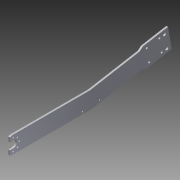
# Autodesk Inventor part: Arm_Link_1
Saved by Autodesk Inventor 2013 (Build 170138000, 138)
## iProperties
Created: 2014-05-15
Part Number: Arm_Link_1
Material: アルミニウム 6061
Document SubType Name: Modeling
Designer: andou
Density: 2.71 g/cm^3
Mass: 19.3291 g
Surface Area: 81.331 cm^2
Volume: 7.13251 cm^3
Author: andou
Autodesk Inventor part; units mm, degrees
ref_plane "YZ Plane" through (0, 0, 0) normal (1, 0, 0) x (0, 1, 0)
ref_plane "XZ Plane" through (0, 0, 0) normal (0, 1, 0) x (-1, 0, 0)
ref_plane "XY Plane" through (0, 0, 0) normal (0, 0, 1) x (1, 0, 0)
sketch "スケッチ2" plane through (0, 0, 0) normal (1, 0, 0) x (0, 1, 0)
  line L0 (0, 0) -> (-89.4689, 0)
  line L1 (-89.4689, -20) -> (1.7498, -20)
  line L2 (0, 0) -> (88.1097, 15.5361)
  line L3 (91.5826, -4.16) -> (1.7498, -20)
  arc A0 (92.1939, 15.4085) -> (88.1097, 15.5361) centre (89.8461, 5.688) ccw
  arc A1 (91.5826, -4.16) -> (95.3769, -2.6433) centre (89.8461, 5.688) ccw
  arc A2 (-93.4689, -19.1652) -> (-89.4689, -20) centre (-89.4689, -10) ccw
  arc A3 (-89.4689, 0) -> (-93.4689, -0.8348) centre (-89.4689, -10) ccw
  arc A4 (-89.4689, -14) -> (-89.4689, -6) centre (-89.4689, -10) ccw
  line L4 (-89.4689, -6) -> (-93.4689, -6)
  line L5 (-89.4689, -14) -> (-93.4689, -14)
  line L6 (-93.4689, -0.8348) -> (-93.4689, -6)
  line L7 (-93.4689, -14) -> (-93.4689, -19.1652)
  line L8 (92.1939, 15.4085) -> (93.0908, 10.3219)
  line L9 (94.48, 2.4434) -> (95.3769, -2.6433)
  line L10 (1.7498, -20) -> (0, 0)
  line L11 (93.0908, 10.3219) -> (94.48, 2.4434)
  dimension "d21" = 20
  dimension "d22" = 10
  dimension "d23" = 170
  dimension "d25" = 10
  dimension "d27" = 10
  dimension "d31" = 8
  dimension "d33" = 4
  dimension "d35" = 4
  dimension "d36" = 180
  constraints: 24 end point, 10 point on circle, 8 perpendicular, 5 centre point, 4 equal length, 3 equal radius, 2 parallel, 2 tangent, 1 coincident, 1 collinear, 1 horizontal
  measures "d21" distance between parallel lines of L0 L1
  measures "d22" distance from line of L0 A2.centre
  measures "d23" angle of L0 L2
  measures "d25" distance from line of L3 A0.centre
  measures "d27" radius of A3
  measures "d31" diameter of A4
  measures "d33" distance from line of L6 A2.centre
  measures "d35" distance from line of L8 L2.end
  measures "d36" distance of A2.centre A0.centre
extrude "押し出し1" add sketch "スケッチ2" along normal blind 2
sketch "スケッチ4" plane through (0, 0, 0) normal (-1, 0, 0) x (0, 0, 1)
  line L0 (-20, 1.7498) -> (-4.16, 91.5826) projected
  line L1 (-20, -89.4689) -> (-20, 1.7498) projected
  circle A0 centre (-17, -8.5509) radius 1
  circle A1 centre (-15.2569, 11.373) radius 1
  line L2 (-17, -8.5509) -> (-15.2569, 11.373)
  dimension "d57" = 2
  dimension "d59" = 20
  dimension "d60" = 175
  dimension "d61" = 3
  dimension "d62" = 3
  constraints: 2 centre point, 2 end point, 1 equal radius
  measures "d57" diameter of A0
  measures "d59" distance of L2.start L2.end
  measures "d60" angle of L1 L2
  measures "d61" distance from line of L1 L2.start
  measures "d62" distance from line of L0 L2.end
hole "穴2" at (0, -8.5509, -17) at (0, 11.373, -15.2569) direction (1, 0, 0) diameter 1.6 end through all
sketch "スケッチ6" plane through (2, 0, 0) normal (1, 0, 0) x (0, 0, -1)
  line L0 (20, 1.7498) -> (4.16, 91.5826) projected
  arc A0 (4.16, 91.5826) -> (2.6433, 95.3769) centre (-5.688, 89.8461) ccw projected
  line L1 (2.6433, 95.3769) -> (-15.4085, 92.1939) projected
  arc A1 (-15.4085, 92.1939) -> (-15.5361, 88.1097) centre (-5.688, 89.8461) ccw projected
  line L2 (-15.5361, 88.1097) -> (0, 0) projected
  line L3 (-10.2693, 58.2403) -> (-13.4833, 62.0705)
  line L4 (-15.4085, 92.1939) -> (-18.6927, 91.6148)
  line L5 (-18.6927, 91.6148) -> (-13.4833, 62.0705)
  line L6 (2.6433, 95.3769) -> (5.9275, 95.956)
  line L7 (5.9275, 95.956) -> (11.1369, 66.4117)
  line L8 (11.1369, 66.4117) -> (9.4268, 61.7133)
  dimension "d75" = 150
  dimension "d76" = 150
  dimension "d77" = 2.5
  dimension "d78" = 2.5
  dimension "d79" = 30
  constraints: 12 end point, 3 parallel, 2 collinear, 2 point on line
  measures "d75" angle of L2 L3
  measures "d76" angle of L0 L8
  measures "d77" distance between parallel lines of L0 L7
  measures "d78" distance between parallel lines of L2 L5
  measures "d79" distance of L4.end L3.end
extrude "押し出し2" add sketch "スケッチ6" against normal blind 2
sketch "スケッチ5" plane through (2, 0, 0) normal (1, 0, 0) x (0, 0, -1)
  line L0 (2.6433, 95.3769) -> (-15.4085, 92.1939) projected
  circle A0 centre (-13.3928, 87.4722) radius 1.5
  circle A1 centre (2.3641, 90.2505) radius 1.5
  line L1 (-13.4833, 62.0705) -> (-18.6927, 91.6148) projected
  line L2 (-18.6927, 91.6148) -> (5.9275, 95.956) projected
  line L3 (5.9275, 95.956) -> (11.1369, 66.4117) projected
  line L4 (11.1369, 66.4117) -> (9.4268, 61.7133) projected
  line L5 (9.4268, 61.7133) -> (20, 1.7498) projected
  line L6 (20, 1.7498) -> (20, -89.4689) projected
  arc A2 (19.1652, -93.4689) -> (20, -89.4689) centre (10, -89.4689) ccw projected
  line L7 (19.1652, -93.4689) -> (14, -93.4689) projected
  line L8 (14, -93.4689) -> (14, -89.4689) projected
  arc A3 (14, -89.4689) -> (6, -89.4689) centre (10, -89.4689) ccw projected
  line L9 (6, -89.4689) -> (6, -93.4689) projected
  line L10 (6, -93.4689) -> (0.8348, -93.4689) projected
  arc A4 (0, -89.4689) -> (0.8348, -93.4689) centre (10, -89.4689) ccw projected
  line L11 (0, -89.4689) -> (0, 0) projected
  line L12 (0, 0) -> (-10.2693, 58.2403) projected
  line L13 (-10.2693, 58.2403) -> (-13.4833, 62.0705) projected
  circle A5 centre (17, -8.5509) radius 0.8 projected
  circle A6 centre (15.2569, 11.373) radius 0.8 projected
  dimension "d70" = 5
  dimension "d71" = 5
  dimension "d72" = 3
  dimension "d114" = 16
  dimension "d123" = 4.5
  constraints: 2 centre point, 1 equal radius
  measures "d70" distance from line of L0 A0.centre
  measures "d71" distance from line of L0 A1.centre
  measures "d72" diameter of A1
  measures "d114" distance of A1.centre A0.centre
  measures "d123" distance from line of L1 A0.centre
hole "穴3" at (2, 87.4722, 13.3928) at (2, 90.2505, -2.3641) direction (-1, 0, 0) diameter 4 end through all
sketch "スケッチ7" plane through (2, 0, 0) normal (1, 0, 0) x (0, 0, -1)
  arc A0 (0, -89.4689) -> (0.8348, -93.4689) centre (10, -89.4689) ccw projected
  line L0 (0.8348, -93.4689) -> (6, -93.4689) projected
  circle A1 centre (3, -89.4689) radius 1
  dimension "d89" = 4
  dimension "d90" = 7
  dimension "d91" = 2
  constraints: 1 centre point
  measures "d89" distance from line of L0 A1.centre
  measures "d90" distance of A1.centre A0.centre
  measures "d91" diameter of A1
hole "穴4" at (2, -89.4689, -3) direction (-1, 0, 0) diameter 2 end through all
pattern_circular "円形状パターン3" count 5 over 180 about axis through (0, -89.4689, -10) along (-1, 0, 0) of "穴4"
sketch "スケッチ8" plane through (2, 0, 0) normal (1, 0, 0) x (0, 0, -1)
  line L0 (5.9275, 95.956) -> (-18.6927, 91.6148) projected
  line L1 (-18.6927, 91.6148) -> (-13.4833, 62.0705) projected
  circle A0 centre (-12.351, 81.5633) radius 1.5
  circle A1 centre (3.406, 84.3417) radius 1.5
  dimension "d102" = 11
  dimension "d103" = 11
  dimension "d104" = 16
  dimension "d105" = 4.5
  dimension "d106" = 3
  constraints: 2 centre point, 1 equal radius
  measures "d102" distance from line of L0 A0.centre
  measures "d103" distance from line of L0 A1.centre
  measures "d104" distance of A1.centre A0.centre
  measures "d105" distance from line of L1 A0.centre
  measures "d106" diameter of A1
hole "穴5" at (2, 81.5633, 12.351) at (2, 84.3417, -3.406) direction (-1, 0, 0) diameter 2.5 end through all
sketch "スケッチ11" plane through (2, 0, 0) normal (1, 0, 0) x (0, 0, -1)
  circle A0 centre (-12.351, 81.5633) radius 1.25 projected
  circle A1 centre (3.406, 84.3417) radius 1.25 projected
  line L0 (-18.6927, 91.6148) -> (-13.4833, 62.0705) projected
  circle A2 centre (-9.7462, 66.7912) radius 1.5
  circle A3 centre (6.0107, 69.5696) radius 1.5
  dimension "d124" = 3
  dimension "d126" = 16
  dimension "d127" = 15
  dimension "d128" = 4.5
  dimension "d130" = 15
  constraints: 2 centre point, 1 equal radius
  measures "d124" diameter of A2
  measures "d126" distance of A3.centre A2.centre
  measures "d127" distance of A0.centre A2.centre
  measures "d128" distance from line of L0 A2.centre
  measures "d130" distance of A1.centre A3.centre
hole "穴6" at (2, 66.7912, 9.7462) at (2, 69.5696, -6.0107) direction (-1, 0, 0) diameter 2.5 end through all
